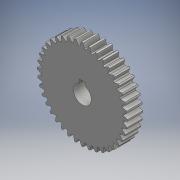
# Autodesk Inventor part: gear_big
Saved by Autodesk Inventor 2016 (Build 200138000, 138)
## iProperties
Created: 2015-10-28
Part Number: gear_big
Material: Generic
Document SubType Name: Modeling
Designer: Meet
Density: 1 g/cm^3
Appearance: Default
Author: Meet
Autodesk Inventor part; units mm, degrees
ref_plane "YZ Plane" through (0, 0, 0) normal (1, 0, 0) x (0, 1, 0)
ref_plane "XZ Plane" through (0, 0, 0) normal (0, 1, 0) x (-1, 0, 0)
ref_plane "XY Plane" through (0, 0, 0) normal (0, 0, 1) x (1, 0, 0)
sketch "Sketch1" plane through (0, 0, 0) normal (0, 1, 0) x (-1, 0, 0)
  arc A0 (43.993, -0.7854) -> (43.993, 0.7854) centre (0, 0) ccw
  arc A1 (39.9306, 2.3548) -> (39.9306, -2.3548) centre (0, 0) ccw
  line L0 (0, 0) -> (40, 0) construction
  line L1 (0, 0) -> (44, 0) construction
  line L2 (39.9306, 2.3548) -> (43.993, 0.7854)
  line L3 (39.9306, -2.3548) -> (43.993, -0.7854)
  constraints: 8 end point, 4 point on circle, 2 centre point, 2 coincident, 2 horizontal, 2 symmetric about line, 1 point on line
extrude "Extrusion1" add sketch "Sketch1" along normal blind 15
pattern_circular "Circular Pattern1" count 40 over 360 about axis through (0, 0, 0) along (0, 1, 0) of "Extrusion1"
sketch "Sketch2" plane through (0, 0, 0) normal (0, -1, 0) x (1, 0, 0)
  line L0 (-3, 8.1131) -> (-3, 11.6631)
  line L1 (3, 8.1131) -> (3, 11.6631)
  line L2 (-3, 11.6631) -> (3, 11.6631)
  arc A0 (-3, 8.1131) -> (3, 8.1131) centre (0, 0) ccw
  constraints: 6 end point, 2 point on circle, 1 centre point, 1 coincident, 1 horizontal, 1 vertical
extrude "Extrusion2" cut sketch "Sketch2" against normal blind 15
body "Solid1"
